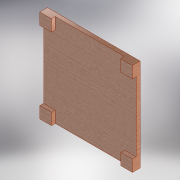
# Autodesk Inventor part: WoodBase
Saved by Autodesk Inventor 2018.2 (Build 222227000, 227)
## iProperties
Created: 2018-03-28
Part Number: WoodBase
Material: Wood (Oak)
Document SubType Name: Modeling
Designer: Muchen He
Density: 0.76 g/cm^3
Appearance: White Oak - Natural Medium Gloss
Author: Muchen He
Autodesk Inventor part; units mm, degrees
ref_plane "YZ Plane" through (0, 0, 0) normal (1, 0, 0) x (0, 1, 0)
ref_plane "XZ Plane" through (0, 0, 0) normal (0, 1, 0) x (-1, 0, 0)
ref_plane "XY Plane" through (0, 0, 0) normal (0, 0, 1) x (1, 0, 0)
sketch "Sketch1" plane through (0, 0, 0) normal (0, 1, 0) x (-1, 0, 0)
  line L0 (0, 0) -> (-304.8, 0)
  line L1 (-304.8, 0) -> (-304.8, -304.8)
  line L2 (-304.8, -304.8) -> (0, -304.8)
  line L3 (0, -304.8) -> (0, 0)
  dimension "d0" = 304.8
  dimension "d1" = 304.8
  constraints: 8 end point, 2 parallel, 1 horizontal, 1 perpendicular
  measures "d0" distance of L2.end L1.end
  measures "d1" distance of L1.end L0.end
extrude "Extrusion1" add sketch "Sketch1" along normal blind 12.7
sketch "Sketch2" plane through (0, 0, 0) normal (0, -1, 0) x (1, 0, 0)
  line L0 (0, 0) -> (304.8, 0) projected
  line L1 (304.8, 0) -> (266.7, 0)
  line L2 (266.7, 0) -> (266.7, -38.1)
  line L3 (266.7, -38.1) -> (304.8, -38.1)
  line L4 (304.8, -38.1) -> (304.8, 0)
  line L5 (304.8, 0) -> (304.8, -304.8) construction
  line L6 (304.8, -152.4) -> (0, -152.4) construction
  line L7 (0, -304.8) -> (0, 0) construction
  line L8 (152.4, 0) -> (152.4, -304.8) construction
  line L9 (304.8, -304.8) -> (0, -304.8) construction
  line L10 (304.8, -304.8) -> (266.7, -304.8)
  line L11 (266.7, -304.8) -> (266.7, -266.7)
  line L12 (266.7, -266.7) -> (304.8, -266.7)
  line L13 (304.8, -266.7) -> (304.8, -304.8)
  line L14 (0, 0) -> (38.1, 0)
  line L15 (38.1, 0) -> (38.1, -38.1)
  line L16 (38.1, -38.1) -> (0, -38.1)
  line L17 (0, -38.1) -> (0, 0)
  line L18 (38.1, -266.7) -> (0, -266.7)
  line L19 (0, -266.7) -> (0, -304.8)
  line L20 (38.1, -304.8) -> (38.1, -266.7)
  line L21 (0, -304.8) -> (38.1, -304.8)
  dimension "d7" = 38.1
  dimension "d8" = 38.1
  constraints: 36 end point, 9 symmetric about line, 4 midpoint, 2 parallel, 1 horizontal, 1 perpendicular
  measures "d7" distance of L3.end L2.end
  measures "d8" distance of L2.end L1.end
extrude "Extrusion2" add sketch "Sketch2" along normal blind 12.7
body "Solid1"
